hourclock_case (Autodesk Fusion 360 design; units mm, degrees)
Autodesk Fusion 360 part; units mm, degrees
sketch "Sketch1" plane through (0, 0, 0) normal (0, 0, 1) x (1, 0, 0)
  line L0 (0, 0) -> (0, 11)
  line L1 (0, 11) -> (11.25, 30)
  line L2 (11.25, 30) -> (11.25, 45)
  line L3 (0, 75) -> (45, 75)
  line L4 (33.75, 45) -> (33.75, 30)
  line L5 (33.75, 30) -> (45, 11)
  line L6 (45, 11) -> (45, 0)
  line L7 (45, 0) -> (0, 0)
  line L8 (11.25, 45) -> (0, 64)
  line L9 (0, 64) -> (0, 75)
  line L10 (45, 75) -> (45, 64)
  line L11 (45, 64) -> (33.75, 45)
  line L12 (-1.8, 76.8) -> (46.8, 76.8)
  line L13 (46.8, 76.8) -> (46.8, 63.5071)
  line L14 (46.8, 63.5071) -> (35.55, 44.5071)
  line L15 (35.55, 44.5071) -> (35.55, 30.4929)
  line L16 (35.55, 30.4929) -> (46.8, 11.4929)
  line L17 (46.8, 11.4929) -> (46.8, -1.8)
  line L18 (46.8, -1.8) -> (-1.8, -1.8)
  line L19 (-1.8, -1.8) -> (-1.8, 11.4929)
  line L20 (-1.8, 11.4929) -> (9.45, 30.4929)
  line L21 (9.45, 30.4929) -> (9.45, 44.5071)
  line L22 (9.45, 44.5071) -> (-1.8, 63.5071)
  line L23 (-1.8, 63.5071) -> (-1.8, 76.8)
  dimension "d1" = 75
  dimension "d2" = 45
  dimension "d3" = 45
  dimension "d4" = 11
  dimension "d5" = 11
  dimension "d7" = 30
  dimension "d8" = 30
  dimension "d9" = 30
  dimension "d10" = 30
  dimension "d13" = 11.25
  dimension "d14" = 90
  dimension "d15" = 11
  dimension "d16" = 11
  dimension "d17" = 11.25
  dimension "d18" = 11.25
  dimension "d19" = 1.8
  dimension "d20" = 1.8
  dimension "d21" = 1.8
  dimension "d22" = 1.8
  dimension "d24" = 1.8
  dimension "d25" = 1.8
  dimension "d26" = 1.8
  dimension "d27" = 1.8
  dimension "d28" = 1.8
  dimension "d29" = 1.8
  dimension "d30" = 1.8
  dimension "d31" = 1.8
  constraint coincident L0.start L7.end
  constraint vertical L0
  constraint parallel L0 L2
  constraint perpendicular L2 L3
  constraint perpendicular L3 L4
  constraint perpendicular L3 L6
  constraint perpendicular L0 L7
  constraint perpendicular L3 L10
  constraint parallel L3 L12
  constraint perpendicular L12 L13
  constraint perpendicular L12 L15
  constraint parallel L15 L17
  constraint perpendicular L17 L18
  constraint perpendicular L18 L19
  constraint perpendicular L18 L21
  constraint perpendicular L12 L23
  constraint parallel L11 L14
  constraint parallel L5 L16
  constraint parallel L8 L22
  constraint parallel L1 L20
  measures "d1" distance of L3 L7
  measures "d2" distance of L3.start L3.end
  measures "d3" distance of L0.start L6.end
  measures "d4" distance of L0.start L0.end
  measures "d5" distance of L5.end L6.end
  measures "d7" distance of L2.end L3
  measures "d8" vertical distance of L3.end L4.start
  measures "d9" distance of L1.end L7
  measures "d10" distance of L4.end L7
  measures "d13" distance of L3.end L4
  measures "d14" angle of L3 L9
  measures "d15" distance of L3.start L8.end
  measures "d16" distance of L3.end L10.end
  measures "d17" distance of L2 L9
  measures "d18" distance of L0 L2 L7.end
  measures "d19" distance of L3 L12
  measures "d20" distance of L9 L23
  measures "d21" distance of L10 L13
  measures "d22" distance of L4 L15
  measures "d24" distance of L11 L14
  measures "d25" distance of L5 L16
  measures "d26" distance of L7 L18
  measures "d27" distance of L6 L17
  measures "d28" distance of L0 L19
  measures "d29" distance of L2 L21
  measures "d30" distance of L1 L20
  measures "d31" distance of L8 L22
extrude "Extrude1" add sketch "Sketch1" along normal blind 17
sketch "Sketch2" plane through (0, 0, 17) normal (0, 0, 1) x (-1, 0, 0)
  line L0 (-45, -75) -> (-45, -64)
  line L1 (-45, -64) -> (-33.75, -45)
  line L2 (-33.75, -45) -> (-33.75, -30)
  line L3 (-33.75, -30) -> (-45, -11)
  line L4 (-45, -11) -> (-45, 0)
  line L5 (-45, 0) -> (0, 0)
  line L6 (0, 0) -> (0, -11)
  line L7 (0, -11) -> (-11.25, -30)
  line L8 (-11.25, -30) -> (-11.25, -45)
  line L9 (-11.25, -45) -> (0, -64)
  line L10 (0, -64) -> (0, -75)
  line L11 (0, -75) -> (-45, -75)
  line L12 (1.8, -63.5071) -> (-9.45, -44.5071)
  line L13 (-9.45, -44.5071) -> (-9.45, -30.4929)
  line L14 (-9.45, -30.4929) -> (1.8, -11.4929)
  line L15 (1.8, -11.4929) -> (1.8, 1.8)
  line L16 (1.8, 1.8) -> (-46.8, 1.8)
  line L17 (-46.8, 1.8) -> (-46.8, -11.4929)
  line L18 (-46.8, -11.4929) -> (-35.55, -30.4929)
  line L19 (-35.55, -30.4929) -> (-35.55, -44.5071)
  line L20 (-35.55, -44.5071) -> (-46.8, -63.5071)
  line L21 (-46.8, -63.5071) -> (-46.8, -76.8)
  line L22 (-46.8, -76.8) -> (1.8, -76.8)
  line L23 (1.8, -76.8) -> (1.8, -63.5071)
  line L24 (1.8, -76.8) -> (1.8, -63.5071)
  line L25 (-9.45, -44.5071) -> (-9.45, -30.4929)
  line L26 (1.8, -11.4929) -> (1.8, 1.8)
  line L27 (-46.8, 1.8) -> (-46.8, -11.4929)
  line L28 (-35.55, -30.4929) -> (-35.55, -44.5071)
  line L29 (-46.8, -63.5071) -> (-46.8, -76.8)
  constraint coincident L22.end L23.start
  constraint coincident L12.start L23.end
  constraint coincident L12.end L13.start
  constraint coincident L13.end L14.start
  constraint coincident L14.end L15.start
  constraint coincident L15.end L16.start
  constraint coincident L16.end L17.start
  constraint coincident L17.end L18.start
  constraint coincident L18.end L19.start
  constraint coincident L19.end L20.start
  constraint coincident L20.end L21.start
  constraint coincident L21.end L22.start
extrude "Extrude2" add sketch "Sketch2" along normal blind 1.5 contours L0 L1 L2 L3 L4 L5 L6 L7 L8 L9 L10 L11 | L12 L13 L14 L15 L16 L17 L18 L19 L20 L21 L22 L23 L24 L25 L26 L27 L28 L29
sketch "Sketch3" plane through (0, 0, 17) normal (0, 0, -1) x (1, 0, 0)
  line L0 (0, -75) -> (45, -75)
  line L1 (45, -75) -> (45, -64)
  line L2 (45, -64) -> (33.75, -45)
  line L3 (33.75, -45) -> (33.75, -30)
  line L4 (33.75, -30) -> (45, -11)
  line L5 (45, -11) -> (45, 0)
  line L6 (45, 0) -> (0, 0)
  line L7 (0, 0) -> (0, -11)
  line L8 (0, -11) -> (11.25, -30)
  line L9 (11.25, -30) -> (11.25, -45)
  line L10 (11.25, -45) -> (0, -64)
  line L11 (0, -64) -> (0, -75)
  line L12 (8.95, -17.7) -> (16.45, -17.7)
  line L13 (16.45, -17.7) -> (16.45, -26.2)
  line L14 (16.45, -26.2) -> (8.95, -26.2)
  line L15 (8.95, -26.2) -> (8.95, -17.7)
  line L16 (9.45, -30.4929) -> (9.45, -44.5071)
  line L17 (29.55, -16.7) -> (36.55, -16.7)
  line L18 (36.55, -16.7) -> (36.55, -23.7)
  line L19 (36.55, -23.7) -> (29.55, -23.7)
  line L20 (29.55, -23.7) -> (29.55, -16.7)
  line L21 (46.8, 1.8) -> (-1.8, 1.8)
  line L22 (46.8, -11.4929) -> (46.8, 1.8)
  dimension "d37" = 8.5
  dimension "d38" = 7.5
  dimension "d43" = 25.5
  dimension "d44" = 17.25
  dimension "d45" = 7
  dimension "d46" = 7
  dimension "d49" = 0.5
  dimension "d50" = 28
  constraint horizontal L12
  constraint vertical L13
  constraint horizontal L14
  constraint vertical L15
  constraint horizontal L17
  constraint vertical L18
  constraint horizontal L19
  constraint vertical L20
  measures "d37" distance of L12.start L14.end
  measures "d38" distance of L12.start L12.end
  measures "d43" distance of L19 L21
  measures "d44" distance of L20 L22
  measures "d45" distance of L17.end L18.end
  measures "d46" distance of L17.start L17.end
  measures "d49" horizontal distance of L12.start L16.start
  measures "d50" distance of L14 L21
extrude "Extrude3" cut sketch "Sketch3" against normal blind 7 contours L8 L14 L15 | L8 L12 L13 L14 L15 | L17 L18 L19 L20
sketch "Sketch4" plane through (0, 0, 0) normal (0, 0, -1) x (1, 0, 0)
  line L0 (45, -64) -> (45, -75)
  line L1 (45, -75) -> (0, -75)
  line L2 (0, -75) -> (0, -64)
  line L3 (0, -64) -> (11.25, -45)
  line L4 (11.25, -45) -> (11.25, -30)
  line L5 (11.25, -30) -> (0, -11)
  line L6 (0, -11) -> (0, 0)
  line L7 (0, 0) -> (45, 0)
  line L8 (45, 0) -> (45, -11)
  line L9 (45, -11) -> (33.75, -30)
  line L10 (33.75, -30) -> (33.75, -45)
  line L11 (33.75, -45) -> (45, -64)
  line L12 (9.45, -44.5071) -> (-1.8, -63.5071)
  line L13 (-1.8, -63.5071) -> (-1.8, -76.8)
  line L14 (-1.8, -76.8) -> (46.8, -76.8)
  line L15 (46.8, -76.8) -> (46.8, -63.5071)
  line L16 (46.8, -63.5071) -> (35.55, -44.5071)
  line L17 (35.55, -44.5071) -> (35.55, -30.4929)
  line L18 (35.55, -30.4929) -> (46.8, -11.4929)
  line L19 (46.8, -11.4929) -> (46.8, 1.8)
  line L20 (46.8, 1.8) -> (-1.8, 1.8)
  line L21 (-1.8, 1.8) -> (-1.8, -11.4929)
  line L22 (-1.8, -11.4929) -> (9.45, -30.4929)
  line L23 (9.45, -30.4929) -> (9.45, -44.5071)
  line L24 (9.45, -30.4929) -> (11.25, -30.4929)
  line L25 (11.25, -30.4929) -> (11.25, -44.5071)
  line L26 (11.25, -44.5071) -> (9.45, -44.5071)
  line L27 (9.45, -44.5071) -> (9.45, -30.4929)
  line L28 (35.55, -30.4929) -> (33.75, -30.4929)
  line L29 (33.75, -30.4929) -> (33.75, -44.4721)
  line L30 (33.75, -44.4721) -> (35.55, -44.4721)
  line L31 (35.55, -44.4721) -> (35.55, -30.4929)
  constraint horizontal L24
  constraint vertical L25
  constraint horizontal L26
  constraint vertical L27
  constraint coincident L4 L25.end
  constraint coincident L22.end L23.start
  constraint horizontal L28
  constraint vertical L29
  constraint horizontal L30
  constraint vertical L31
  constraint coincident L10 L29.end
  constraint coincident L17.end L18.start
extrude "Extrude4" add sketch "Sketch4" along normal blind 6.5 contours L10 L17 L28 L29 L30 L31 | L4 L23 L24 L25 L26 L27
